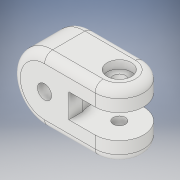
# Autodesk Inventor part: Arm1
Saved by Autodesk Inventor 2017 SP1 (Build 210196100, 196)
## iProperties
Created: 2018-02-11
Part Number: Arm1
Material: ABS Plastic
Document SubType Name: Modeling
Designer: Zach
Density: 1.06 g/cm^3
Appearance: CR White
Author: Zach
Autodesk Inventor part; units mm, degrees
ref_plane "YZ Plane" through (0, 0, 0) normal (1, 0, 0) x (0, 1, 0)
ref_plane "XZ Plane" through (0, 0, 0) normal (0, 1, 0) x (-1, 0, 0)
ref_plane "XY Plane" through (0, 0, 0) normal (0, 0, 1) x (1, 0, 0)
sketch "Sketch2" plane through (0, 0, 0) normal (0, 0, 1) x (1, 0, 0)
  circle A0 centre (0, 0) radius 1.75
  circle A1 centre (0, 0) radius 8 construction
  arc A2 (0, 8) -> (0, -8) centre (0, 0) ccw
  line L0 (0, 8) -> (6, 8)
  line L1 (6, 8) -> (6, -8)
  line L2 (6, -8) -> (0, -8)
  dimension "d0" = 3.5
  dimension "d1" = 16
  dimension "d2" = 6
  constraints: 6 end point, 4 point on circle, 3 centre point, 2 coincident, 2 concentric, 2 horizontal, 2 vertical alignment, 1 perpendicular
  measures "d0" diameter of A0
  measures "d1" diameter of A1
  measures "d2" distance of L0.start L0.end
extrude "Extrusion1" add sketch "Sketch2" along normal blind 12
sketch "Sketch3" plane through (0, -8, 0) normal (0, -1, 0) x (1, 0, 0)
  circle A0 centre (12.5, 6) radius 6 construction
  line L0 (6, 0) -> (6, 12) projected
  line L1 (0, 0) -> (0, 12) projected
  circle A1 centre (12.5, 6) radius 1.5
  arc A2 (12.5, 0) -> (12.5, 12) centre (12.5, 6) ccw
  line L2 (6, 12) -> (12.5, 12)
  line L3 (6, 0) -> (12.5, 0)
  point P0 (6, 6)
  dimension "d5" = 12
  dimension "d6" = 12.5
  dimension "d7" = 3
  constraints: 4 end point, 4 point on circle, 3 centre point, 2 horizontal, 1 coincident, 1 concentric, 1 horizontal alignment, 1 midpoint
  measures "d5" diameter of A0
  measures "d6" distance from line of L1 A0.centre
  measures "d7" diameter of A1
extrude "Extrusion2" add sketch "Sketch3" against normal blind 5
sketch "Sketch4" plane through (0, 8, 0) normal (0, 1, 0) x (1, 0, 0)
  circle A0 centre (12.5, -6) radius 1.5 projected
  line L0 (6, -12) -> (6, 0) projected
  line L1 (6, -12) -> (12.5, -12) projected
  arc A1 (12.5, -12) -> (12.5, 0) centre (12.5, -6) ccw projected
  line L2 (12.5, 0) -> (6, 0) projected
  point P0 (0, 0)
extrude "Extrusion3" add sketch "Sketch4" against normal blind 5
sketch "Sketch6" plane through (0, 8, 12) normal (0, 1, 0) x (1, 0, 0)
  circle A0 centre (12.5, 6) radius 1.5 projected
  circle A1 centre (12.5, 6) radius 3
  point P0 (0, 12)
  dimension "d13" = 6
  constraints: 1 centre point, 1 coincident
  measures "d13" diameter of A1
extrude "Extrusion4" cut sketch "Sketch6" against normal blind 2
sketch "Sketch7" plane through (0, -3, 0) normal (0, 1, 0) x (1, 0, 0)
  arc A0 (12.5, -12) -> (12.5, 0) centre (12.5, -6) ccw projected
  circle A1 centre (12.5, -6) radius 7
  point P0 (0, 0)
  dimension "d16" = 14
  constraints: 1 centre point, 1 coincident
  measures "d16" diameter of A1
extrude "Extrusion5" cut sketch "Sketch7" along normal blind 6
fillet "Fillet1" radius 2 8 edges at (18.5, 8, 6) (6.25, 8, 0) (-8, 0, 0) (6.25, -8, 0) (18.5, -8, 6) (6.25, -8, 12) (-8, 0, 12) (6.25, 8, 12)
body "Solid1"
